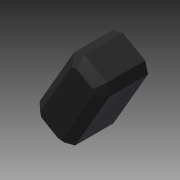
# Autodesk Inventor part: TSOP Holder Straight
Saved by Autodesk Inventor 2015 (Build 190159000, 159)
## iProperties
Created: 2015-11-27
Part Number: TSOP Holder Straight
Material: ABS Plastic
Document SubType Name: Modeling
Designer: James
Density: 1.06 g/cm^3
Appearance: Smooth - White
Author: James
Autodesk Inventor part; units mm, degrees
ref_plane "YZ Plane" through (0, 0, 0) normal (1, 0, 0) x (0, 1, 0)
ref_plane "XZ Plane" through (0, 0, 0) normal (0, 1, 0) x (-1, 0, 0)
ref_plane "XY Plane" through (0, 0, 0) normal (0, 0, 1) x (1, 0, 0)
sketch "Sketch1" plane through (0, 0, 0) normal (0, 1, 0) x (-1, 0, 0)
  line L0 (41.1895, 30.2734) -> (43.9395, 25.5103)
  line L1 (43.9395, 25.5103) -> (47.5768, 27.6103)
  line L2 (42.0768, 37.1366) -> (38.4395, 35.0366)
  line L3 (38.4395, 35.0366) -> (41.1895, 30.2734)
  arc A0 (46.0996, 30.1689) -> (43.5541, 34.578) centre (44.0588, 31.93) ccw
  line L4 (42.0768, 37.1366) -> (43.5541, 34.578)
  line L5 (46.0996, 30.1689) -> (47.5768, 27.6103)
  line L6 (40.2582, 36.0866) -> (43.5582, 36.0866) construction
  circle A1 centre (38.6082, 38.9445) radius 1.4
  line L7 (41.7517, 43.2997) -> (35.9493, 39.9497)
  line L8 (35.9493, 39.9497) -> (35.2173, 37.2177)
  line L9 (39.7286, 29.43) -> (35.2173, 37.2177)
  line L10 (44.4838, 42.5677) -> (41.7517, 43.2997)
  line L11 (44.9838, 41.7016) -> (44.4838, 42.5677)
  line L12 (44.9838, 41.7016) -> (48.976, 34.7869)
  circle A2 centre (47.4248, 23.7248) radius 1.4
  line L13 (52.7668, 24.2851) -> (46.9742, 20.9182)
  line L14 (46.9742, 20.9182) -> (44.24, 21.6423)
  line L15 (39.7286, 29.43) -> (44.24, 21.6423)
  line L16 (53.4908, 27.0193) -> (52.7668, 24.2851)
  line L17 (52.9883, 27.8839) -> (53.4908, 27.0193)
  line L18 (52.9883, 27.8839) -> (48.976, 34.7869)
  point P0 (34.2173, 38.9497)
  point P1 (43.4838, 44.2997)
  point P2 (45.245, 19.9132)
  point P3 (54.4959, 25.2902)
  dimension "d0" = 5
  dimension "d29" = 2.8
  dimension "d32" = 2
  dimension "d33" = 2
  dimension "d34" = 2
  dimension "d35" = 2
  dimension "d41" = 2.8
  constraints: 38 end point, 4 point on line, 3 centre point, 2 point on circle, 1 horizontal, 1 midpoint
  measures "d0" distance of A0.centre L9.start
  measures "d29" diameter of A1
  measures "d32" distance of L7.end point (34.217, 38.95)
  measures "d33" distance of L8.end point (34.217, 38.95)
  measures "d34" distance of L10.start point (43.484, 44.3)
  measures "d35" distance of L7.start point (43.484, 44.3)
  measures "d41" diameter of A2
extrude "Extrusion1" add sketch "Sketch1" along normal blind 12
sketch "Sketch3" plane through (-38.4395, 2, 35.0366) normal (-0.8660254, 0, 0.5) x (0.5, 0, 0.8660254)
  line L0 (-11, 0) -> (0, 0) projected
  line L1 (-5.5, 0) -> (-5.5, 3.3)
  circle A0 centre (-5.5, 3.3) radius 1.65
  point P0 (-11.1228, -2)
  dimension "d20" = 3.3
  dimension "d21" = 3.3
  constraints: 2 end point, 1 centre point, 1 coincident, 1 midpoint, 1 vertical
  measures "d20" distance of L1.start L1.end
  measures "d21" diameter of A0
extrude "Extrusion3" cut sketch "Sketch3" along normal through all
sketch "Sketch4" plane through (0, 0, 0) normal (0, -1, 0) x (1, 0, 0)
  line L0 (-42.0768, 37.1366) -> (-38.4395, 35.0366) projected
  line L1 (-38.4395, 35.0366) -> (-43.9395, 25.5103) projected
  line L2 (-43.9395, 25.5103) -> (-47.5768, 27.6103) projected
  line L3 (-47.5768, 27.6103) -> (-46.0996, 30.1689) projected
  arc A0 (-43.5541, 34.578) -> (-46.0996, 30.1689) centre (-44.0588, 31.93) ccw projected
  line L4 (-43.5541, 34.578) -> (-42.0768, 37.1366) projected
  circle A1 centre (-47.4248, 23.7248) radius 1.4 projected
  circle A2 centre (-38.6082, 38.9445) radius 1.4 projected
  line L5 (-44.24, 21.6423) -> (-35.2173, 37.2177) projected
  line L6 (-35.2173, 37.2177) -> (-35.9493, 39.9497) projected
  line L7 (-35.9493, 39.9497) -> (-41.7517, 43.2997) projected
  line L8 (-41.7517, 43.2997) -> (-44.4838, 42.5677) projected
  line L9 (-44.4838, 42.5677) -> (-48.976, 34.7869) projected
  line L10 (-48.976, 34.7869) -> (-53.4908, 27.0193) projected
  line L11 (-53.4908, 27.0193) -> (-52.7668, 24.2851) projected
  line L12 (-52.7668, 24.2851) -> (-46.9742, 20.9182) projected
  line L13 (-46.9742, 20.9182) -> (-44.24, 21.6423) projected
  point P0 (0, 0)
extrude "Extrusion4" add sketch "Sketch4" against normal blind 2 contours L0 L1 L2 L3 A0 L4 | A1 | A2
chamfer "Chamfer2" distance 2 angle 45 9 edges at (-53.1288, 0, 25.6522) (-51.2334, 0, 30.9031) (-46.7299, 0, 38.6773) (-43.1177, 0, 42.9337) (-38.8505, 0, 41.6247) (-35.5833, 0, 38.5837) (-39.7286, 0, 29.43) (-45.6071, 0, 21.2803) (-49.8705, 0, 22.6017)
equation "\"d33\" = d32"
equation "\"d35\" = d34"
body "Solid1"
